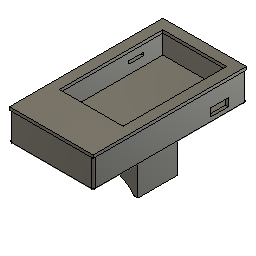
雷达支架 (Autodesk Fusion 360 design; units mm, degrees)
Autodesk Fusion 360 part; units mm, degrees
sketch "草图1" plane through (0, 0, 0) normal (0, 1, 0) x (1, 0, 0)
  line L0 (0, 0) -> (42, 0)
  line L1 (42, 0) -> (42, 77)
  line L2 (42, 77) -> (0, 77)
  line L3 (0, 77) -> (0, 0)
  line L4 (1.5, 1.5) -> (40.5, 1.5)
  line L5 (40.5, 1.5) -> (40.5, 75.5)
  line L6 (40.5, 75.5) -> (1.5, 75.5)
  line L7 (1.5, 75.5) -> (1.5, 1.5)
  line L8 (6, 28.5) -> (36, 28.5)
  line L9 (36, 28.5) -> (36, 48.5)
  line L10 (36, 48.5) -> (6, 48.5)
  line L11 (6, 48.5) -> (6, 28.5)
  dimension "d1" = 42
  dimension "d2" = 77
  dimension "d3" = -1.5
  dimension "d12" = 30
  dimension "d13" = 20
  dimension "d14" = 6
  dimension "d15" = 28.5
  constraint horizontal L0
  constraint vertical L1
  constraint horizontal L2
  constraint vertical L3
  constraint coincident L0.start L3.end
  constraint horizontal L8
  constraint vertical L9
  constraint horizontal L10
  constraint vertical L11
  measures "d1" distance of L0.start L0.end
  measures "d2" distance of L0.start L2.end
  measures "d12" distance of L8.start L8.end
  measures "d13" distance of L8.start L10.end
  measures "d14" distance of L3 L11
  measures "d15" distance of L2 L10
extrude "拉伸1" add sketch "草图1" along normal blind 1.5 contours L0 L1 L2 L3 | L4 L5 L6 L7 | L8 L9 L10 L11 makes body 1
extrude "拉伸2" add sketch "草图1" along normal blind 14.5 contours L0 L1 L2 L3 bodies 1
sketch "草图2" plane through (0, 14.5, 0) normal (0, 1, 0) x (-1, 0, 0)
  line L0 (-1.5, -1.5) -> (-1.5, -75.5)
  line L1 (-1.5, -75.5) -> (-40.5, -75.5)
  line L2 (-40.5, -75.5) -> (-40.5, -1.5)
  line L3 (-40.5, -1.5) -> (-1.5, -1.5)
  line L4 (0, -77) -> (0, 0)
  line L5 (0, 0) -> (-42, 0)
  line L6 (-42, 0) -> (-42, -77)
  line L7 (-42, -77) -> (0, -77)
  line L8 (0, 0) -> (-42, 0)
  line L9 (-42, 0) -> (-42, -77)
  line L10 (-42, -77) -> (0, -77)
  line L11 (0, -77) -> (0, 0)
  line L12 (-37, -20) -> (-37, -72)
  line L13 (-37, -72) -> (-5, -72)
  line L14 (-5, -72) -> (-5, -20)
  line L15 (-5, -20) -> (-37, -20)
  constraint horizontal L8
  constraint vertical L9
  constraint horizontal L10
  constraint vertical L11
  constraint coincident L6.end L7.start
  constraint coincident L4.end L5.start
  constraint perpendicular L12 L15
extrude "拉伸3" add sketch "草图2" along normal blind 1.5 separate body contours L0 L1 L2 L3 | L4 L5 L6 L7 L8 L9 L10 L11 makes body 2
copy_body "实体->零部件1" bodies 2 removing the originals makes body 3 in component "Component'"
extrude "拉伸4" add sketch "草图1" against normal blind 30 contours L8 L9 L10 L11 bodies 1
sketch "草图3" plane through (0, 0, -48.5) normal (0, 0, -1) x (-1, 0, 0)
  line L0 (-6, 0) -> (-36, 0)
  line L1 (-36, 0) -> (-36, -30)
  line L2 (-36, -30) -> (-6, -30)
  line L3 (-6, -30) -> (-6, 0)
  circle A0 centre (-21, -30) radius 16.5
  line L4 (-6, -20) -> (-36, -20)
  line L5 (-42, 0) -> (0, 0)
  dimension "d18" = 33
  dimension "d19" = 20
  constraint midpoint L2 A0.centre
  constraint coincident L3 L4.start
  constraint coincident L1 L4.end
  constraint perpendicular L1 L4
  measures "d18" diameter of A0
  measures "d19" distance of L4 L5
extrude "拉伸5" cut sketch "草图3" against normal blind 40 contours L3 A0 L4 | L1 A0 L4 | L1 L2 L3 A0 L4 | A0 L4 bodies 1
sketch "草图4" plane through (42, 0, 0) normal (1, 0, 0) x (0, 0, -1)
  line L0 (0, 0) -> (77, 0)
  line L1 (77, 0) -> (77, 14.5)
  line L2 (77, 14.5) -> (0, 14.5)
  line L3 (0, 14.5) -> (0, 0)
  line L4 (68, 3) -> (59, 3)
  line L5 (59, 3) -> (59, 7)
  line L6 (59, 7) -> (68, 7)
  line L7 (68, 7) -> (68, 3)
  line L8 (0, 0) -> (77, 0)
  dimension "d22" = 9
  dimension "d23" = 4
  dimension "d24" = 3
  dimension "d25" = 9
  constraint horizontal L4
  constraint vertical L5
  constraint horizontal L6
  constraint vertical L7
  measures "d22" distance of L4.start L4.end
  measures "d23" distance of L4.start L6.end
  measures "d24" distance of L4 L8
  measures "d25" distance of L1 L7
extrude "拉伸6" cut sketch "草图4" against normal blind 10 contours L4 L5 L6 L7 bodies 1
sketch "草图5" plane through (0, 0, 0) normal (-1, 0, 0) x (0, 0, 1)
  line L0 (-77, 0) -> (0, 0)
  line L1 (0, 0) -> (0, 14.5)
  line L2 (0, 14.5) -> (-77, 14.5)
  line L3 (-77, 14.5) -> (-77, 0)
  line L4 (-58.5, 6) -> (-66, 6)
  line L5 (-66, 6) -> (-66, 7.5)
  line L6 (-66, 7.5) -> (-58.5, 7.5)
  line L7 (-58.5, 7.5) -> (-58.5, 6)
  line L8 (-77, 0) -> (0, 0)
  dimension "d28" = 7.5
  dimension "d29" = 1.5
  dimension "d30" = 11
  dimension "d31" = 6
  constraint horizontal L4
  constraint vertical L5
  constraint horizontal L6
  constraint vertical L7
  measures "d28" distance of L4.start L4.end
  measures "d29" distance of L4.end L5.end
  measures "d30" distance of L3 L5
  measures "d31" distance of L4 L8
extrude "拉伸7" cut sketch "草图5" against normal blind 4 contours L4 L5 L6 L7 bodies 1
fillet "圆角1" radius 1 8 edges at (0, 7.25, 0) (0, 0, -38.5) (21, 0, 0) (42, 7.25, 0) (42, 0, -38.5) (42, 7.25, -77) (21, 0, -77) (0, 7.25, -77) on bodies 1
copy_body "实体->零部件2" bodies 1 removing the originals makes body 4 in component "Component''"
component "Component'" placed x (1, 0, 0) y (0, 1, 0) z (0, 0, 1) at (-74.4932, -11.3757, 63.999)
component "Component''" placed x (1, 0, 0) y (0, 1, 0) z (0, 0, 1) at (-74.4932, -11.3757, 63.999)
